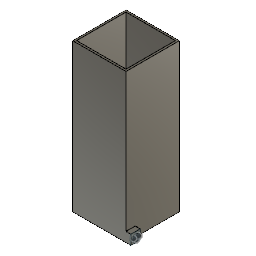
FRASCO COM FURO (Autodesk Fusion 360 design; units mm, degrees)
Autodesk Fusion 360 part; units mm, degrees
sketch "Esboço1" plane through (0, 0, 0) normal (0, 0, 1) x (1, 0, 0)
  line L0 (20, 20) -> (76, 20)
  line L1 (76, 20) -> (76, 76)
  line L2 (76, 76) -> (20, 76)
  line L3 (20, 76) -> (20, 20)
  dimension "d1" = 56
  dimension "d2" = 56
  constraint horizontal L0
  constraint vertical L1
  constraint horizontal L2
  constraint vertical L3
  measures "d1" distance of L0.start L0.end
  measures "d2" distance of L0.start L2.end
extrude "Extrusão1" add sketch "Esboço1" along normal blind 150
shell "Casca1" thickness 3 removed faces 1 at (38.6667, 57.3333, 150)
sketch "Esboço2" plane through (76, 0, 0) normal (1, 0, 0) x (0, 1, 0)
  line L0 (20, 0) -> (76, 0)
  line L1 (76, 0) -> (76, 150)
  line L2 (76, 150) -> (20, 150)
  line L3 (20, 150) -> (20, 0)
  line L4 (20, 0) -> (23, 0)
  line L5 (23, 0) -> (23, 3)
  line L6 (23, 3) -> (26, 3)
  line L7 (26, 3) -> (26, 5.5)
  circle A0 centre (26, 5.5) radius 2.5
  line L8 (20, 0) -> (30.3858, 0)
  line L9 (30.3858, 0) -> (30.3858, 10)
  line L10 (30.3858, 10) -> (20, 10)
  dimension "d6" = 3
  dimension "d7" = 3
  dimension "d8" = 3
  dimension "d9" = 2.5
  dimension "d10" = 5
  constraint coincident L0.start L3.end
  constraint perpendicular L3 L4
  constraint perpendicular L0 L5
  constraint perpendicular L5 L6
  constraint perpendicular L6 L7
  constraint coincident L7.end A0.centre
  constraint coincident L0 L8.end
  constraint perpendicular L3 L8
  constraint perpendicular L0 L9
  constraint coincident L3 L10.end
  constraint perpendicular L3 L10
  measures "d6" distance of L0.start L4.end
  measures "d7" distance of L4.end L5.end
  measures "d8" distance of L5.end L6.end
  measures "d9" distance of L6.end L7.end
  measures "d10" diameter of A0
extrude "Extrusão2" add sketch "Esboço2" along normal blind 4 contours L0 L3 L4 L8 L9 L10
move_face "Deslocar faces1" offset -3 1 faces at (76, 26.6109, 4.9332)
sketch "Esboço3" plane through (80, 0, 0) normal (1, 0, 0) x (0, 1, 0)
  circle A0 centre (26, 5.5) radius 2.5
  line L0 (30.3858, 10) -> (20, 10)
  line L1 (20, 10) -> (20, 0)
  line L2 (20, 0) -> (30.3858, 0)
  line L3 (30.3858, 0) -> (30.3858, 10)
  circle A1 centre (26, 3) radius 2
  line L4 (28.4495, 5) -> (27.9596, 2.6)
  line L5 (24.0404, 2.6) -> (23.5505, 5)
  constraint coincident A0 A1.centre
  constraint coincident A0 L4.start
  constraint coincident A1 L4.end
  constraint tangent A1 L4
  constraint coincident A1 L5.start
  constraint coincident A0 L5.end
  constraint tangent A0 L5
move_face "Deslocar faces2" offset -1 4 faces at (20, 57.3333, 50) (57.3333, 76, 100) (38.6667, 20, 53.3333) (76, 42.1286, 103.3333)
